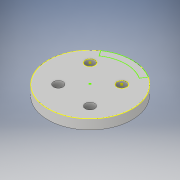
# Autodesk Inventor part: mount_interface
Saved by Autodesk Inventor 2019 (Build 230136000, 136)
## iProperties
Created: 2019-03-09
Part Number: mount_interface
Material: Generic
Document SubType Name: Modeling
Designer: Jaden
Density: 1 g/cm^3
Appearance: Default
Author: Jaden
Autodesk Inventor part; units mm, degrees
ref_plane "YZ Plane" through (0, 0, 0) normal (1, 0, 0) x (0, 1, 0)
ref_plane "XZ Plane" through (0, 0, 0) normal (0, 1, 0) x (-1, 0, 0)
ref_plane "XY Plane" through (0, 0, 0) normal (0, 0, 1) x (1, 0, 0)
sketch "Sketch1" plane through (0, 0, 0) normal (0, 1, 0) x (-1, 0, 0)
  circle A0 centre (-6.7175, 6.7175) radius 1.7
  circle A1 centre (5.6568, 5.6568) radius 1.7
  circle A2 centre (6.7175, -6.7175) radius 1.7
  circle A3 centre (-5.6569, -5.6569) radius 1.7
  line L0 (0, 0) -> (-10.6066, 10.6066) construction
  arc A4 (14.1421, 5) -> (14.1421, -5) centre (0, 0) ccw
  line L1 (0, 0) -> (15, 0) construction
  line L2 (0, 0) -> (10.6066, -10.6066) construction
  line L3 (0, 0) -> (15, 0) construction
  line L4 (0, 0) -> (-10.6066, -10.6066) construction
  line L5 (0, 0) -> (10.6066, 10.6066) construction
  line L6 (0, 0) -> (15, 0) construction
  circle A5 centre (0, 0) radius 15
  dimension "d0" = 3.4
  dimension "d1" = 3.4
  dimension "d2" = 3.4
  dimension "d3" = 3.4
  dimension "d4" = 135
  dimension "d5" = 45
  dimension "d6" = 45
  dimension "d7" = 11.3137
  dimension "d8" = 5.6569
  dimension "d9" = 13.435
  dimension "d10" = 6.7175
  dimension "d14" = 30
  constraints: 14 end point, 6 centre point, 6 point on circle, 4 point on line, 3 equal length, 3 horizontal, 1 perpendicular
  measures "d0" diameter of A0
  measures "d1" diameter of A1
  measures "d2" diameter of A2
  measures "d3" diameter of A3
  measures "d4" angle of L1 L0
  measures "d5" angle of L2 L3
  measures "d6" angle of L6 L5
  measures "d7" horizontal distance of A3.centre A1.centre
  measures "d8" horizontal distance of L0.start A3.centre
  measures "d9" horizontal distance of A0.centre A2.centre
  measures "d10" horizontal distance of A0.centre L0.start
  measures "d14" diameter of A5
extrude "Extrusion1" add sketch "Sketch1" along normal blind 3.5
sketch "Sketch3" plane through (0, 3.5, 0) normal (0, 1, 0) x (1, 0, 0)
  circle A0 centre (-6.7175, 6.7175) radius 1.7 projected
  circle A1 centre (5.6569, 5.6569) radius 1.7 projected
  circle A2 centre (0, 0) radius 15 projected
  arc A3 (8.0924, 12.6453) -> (-8.5504, 12.3244) centre (0.0125, -0.0399) ccw
  arc A4 (6.8579, 10.707) -> (-7.2223, 10.4172) centre (0.0353, -0.0047) ccw
  line L0 (-7.2223, 10.4172) -> (-8.5504, 12.3244)
  line L1 (6.8579, 10.707) -> (8.0924, 12.6453)
  point P0 (0.0353, -0.0047)
  constraints: 4 end point, 4 point on circle, 2 centre point, 2 tangent, 2 other
body "Solid1"
